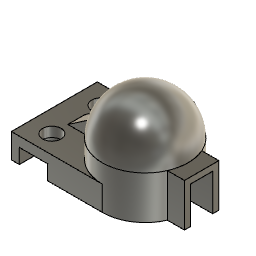
drawing_8 v1 (Autodesk Fusion 360 design; units mm, degrees)
Autodesk Fusion 360 part; units mm, degrees
box "BoxPrimitive1" add length 70 width 74 height 20 placed x (0, -1, 0) y (1, 0, 0) z (0, 0, 1) at (-30, 30, 0)
sketch "Sketch2" plane through (0, 0, 20) normal (0, 0, 1) x (-1, 0, 0)
  line L0 (30, 40) -> (-44, 40)
  line L1 (-44, 40) -> (-44, -30)
  line L2 (-44, -30) -> (30, -30)
  line L3 (30, -30) -> (30, 40)
  circle A0 centre (12, -15) radius 7.5
  circle A1 centre (12, 25) radius 7.5
  point P0 (30, -15)
  point P1 (30, 25)
  point P2 (12, -30)
  point P3 (12, -15)
  point P4 (12, 25)
  dimension "d9" = 15
  dimension "d10" = 15
  constraint coincident P3 A0.centre
  constraint coincident P4 A1.centre
  measures "d9" diameter of A0
  measures "d10" diameter of A1
extrude "Extrude1" cut sketch "Sketch2" against normal blind 378 contours A0 | A1
sketch "Sketch3" plane through (0, 0, 0) normal (0, 0, -1) x (1, 0, 0)
  circle A0 centre (-12, -15) radius 7.5
  circle A1 centre (-12, 25) radius 7.5
  line L0 (44, 40) -> (-30, 40)
  line L1 (-30, 40) -> (-30, -30)
  line L2 (-30, -30) -> (44, -30)
  line L3 (44, -30) -> (44, 40)
  line L4 (-0.5, 25) -> (-0.5, 40)
  line L5 (-0.5, 40) -> (-23.5, 40)
  line L6 (-23.5, 40) -> (-23.5, 25)
  line L7 (-23.5, -15) -> (-23.5, -30)
  line L8 (-23.5, -30) -> (-0.5, -30)
  line L9 (-0.5, -30) -> (-0.5, -15)
  arc A2 (-0.5, -15) -> (-23.5, -15) centre (-12, -15) ccw
  arc A3 (-23.5, 25) -> (-0.5, 25) centre (-12, 25) ccw
  dimension "d13" = 23
  dimension "d14" = 23
  dimension "d15" = 23
  dimension "d16" = 23
  constraint concentric A1 A3
  constraint concentric A0 A2
  constraint coincident L0 L4.end
  constraint tangent L4 A3
  constraint perpendicular L0 L4
  constraint perpendicular L4 L5
  constraint tangent L7 A2
  constraint coincident L2 L8.end
  constraint tangent L9 A2
  measures "d13" diameter of A3
  measures "d14" diameter of A2
  measures "d15" distance of L4.end L5.end
  measures "d16" distance of L7.end L8.end
extrude "Extrude2" cut sketch "Sketch3" against normal blind 12 contours L0 L4 L5 L6 A3 | L2 L7 L8 L9 A2
sketch "Sketch4" plane through (0, 0, 20) normal (0, 0, 1) x (-1, 0, 0)
  circle A0 centre (12, -15) radius 7.5
  circle A1 centre (12, 25) radius 7.5
  line L0 (30, 40) -> (-44, 40)
  line L1 (-44, -30) -> (30, -30)
  line L2 (30, -30) -> (30, 40)
  circle A2 centre (-44, 5) radius 35
  point P0 (-44, 5)
  constraint coincident P0 A2.centre
  constraint coincident L1.start A2
extrude "Extrude3" add sketch "Sketch4" along normal blind 15 and the other way blind 20 contours A2
sketch "Sketch5" plane through (0, 0, 35) normal (0, 0, 1) x (-1, 0, 0)
  circle A0 centre (-44, 5) radius 35
sketch "Sketch6" plane through (0, 0, 35) normal (0, 0, 1) x (-1, 0, 0)
  circle A0 centre (-44, 5) radius 35
  dimension "d23" = 70
  measures "d23" diameter of A0
sphere "SpherePrimitive1" add diameter 70 placed x (-1, 0, 0) y (0, -1, 0) z (0, 0, 1) at (44, -5, 35)
sketch "Sketch8" plane through (0, 30, 0) normal (0, 1, 0) x (-1, 0, 0)
  line L0 (0.5, 0) -> (0.5, 12)
  line L1 (0.5, 12) -> (23.5, 12)
  line L2 (23.5, 12) -> (23.5, 0)
  line L3 (23.5, 0) -> (30, 0)
  line L4 (30, 0) -> (30, 20)
  line L5 (30, 20) -> (-44, 20)
  line L6 (-44, 20) -> (-44, 0)
  line L7 (-44, 0) -> (0.5, 0)
  line L8 (-34, 50) -> (-54, 50)
  line L9 (-54, 50) -> (-54, 30)
  line L10 (-54, 30) -> (-34, 30)
  line L11 (-34, 30) -> (-34, 50)
  line L12 (-34, 50) -> (-54, 30) construction
  line L13 (-54, 50) -> (-34, 30) construction
  point P0 (-44, 40)
  point P1 (-44, 40)
  dimension "d26" = 20
  dimension "d27" = 20
  constraint horizontal L8
  constraint perpendicular L8 L9
  constraint parallel L8 L10
  constraint parallel L9 L11
  constraint coincident L12 P1
  constraint coincident L13 P1
  constraint coincident P1 P0
  measures "d26" distance of L9.end L10.end
  measures "d27" distance of L8.end L9.end
extrude "Extrude4" cut sketch "Sketch8" against normal blind 15 contours L8 L9 L10 L11
sketch "Sketch9" plane through (0, 0, 0) normal (0, 0, -1) x (1, 0, 0)
  line L0 (44, 40) -> (-0.5, 40)
  line L1 (-0.5, 40) -> (-0.5, 25)
  arc A0 (-23.5, 25) -> (-0.5, 25) centre (-12, 25) ccw
  line L2 (-23.5, 25) -> (-23.5, 40)
  line L3 (-23.5, 40) -> (-30, 40)
  line L4 (-30, 40) -> (-30, -30)
  line L5 (-30, -30) -> (-23.5, -30)
  line L6 (-23.5, -30) -> (-23.5, -15)
  arc A1 (-0.5, -15) -> (-23.5, -15) centre (-12, -15) ccw
  line L7 (-0.5, -15) -> (-0.5, -30)
  line L8 (-0.5, -30) -> (44, -30)
  arc A2 (44, -30) -> (44, 40) centre (44, 5) ccw
  circle A3 centre (44, 5) radius 28
extrude "Extrude5" cut sketch "Sketch9" against normal blind 35 contours A3
sketch "Sketch10" plane through (0, 0, 35) normal (0, 0, -1) x (1, 0, 0)
  line L0 (34, -21.1534) -> (34, -15)
  line L1 (34, -15) -> (54, -15)
  line L2 (54, -15) -> (54, -21.1534)
  arc A0 (54, -21.1534) -> (34, -21.1534) centre (44, 5) ccw
  circle A1 centre (44, 5) radius 28
  constraint concentric A0 A1
sphere "SpherePrimitive2" cut diameter 56 placed x (1, 0, 0) y (0, -1, 0) z (0, 0, -1) at (44, -5, 35)
sketch "Sketch12" plane through (0, 0, 20) normal (0, 0, 1) x (-1, 0, 0)
  arc A0 (-44, -30) -> (-44, 40) centre (-44, 5) ccw
  line L0 (-44, -30) -> (30, -30)
  line L1 (30, -30) -> (30, 40)
  line L2 (30, 40) -> (-44, 40)
  circle A1 centre (12, -15) radius 7.5
  circle A2 centre (12, 25) radius 7.5
  line L3 (12, 5) -> (12, -2)
  line L4 (12, -2) -> (12, 5)
  line L5 (12, 5) -> (12, 12)
  line L6 (12, -2) -> (-11.2915, -2)
  line L7 (-11.2915, -2) -> (-11.2915, 12)
  line L8 (-11.2915, 12) -> (12, 12)
  point P0 (30, 5)
  constraint midpoint L1 P0
  constraint perpendicular L3 L6
  constraint perpendicular L6 L7
  constraint perpendicular L7 L8
extrude "Extrude6" add sketch "Sketch12" along normal blind 15 contours A0 L6 L7 L8 | A0 L3 L4 L5 L6 L8
sketch "Sketch13" plane through (0, 2, 0) normal (0, 1, 0) x (-1, 0, 0)
  line L0 (-9.7071, 35) -> (-9.7071, 20)
  line L1 (-9.7071, 20) -> (12, 20)
  line L2 (12, 20) -> (12, 35)
  line L3 (12, 35) -> (-9.7071, 35)
  line L4 (12, 20) -> (-10, 35)
  constraint coincident L1.end L2.start
extrude "Extrude7" cut sketch "Sketch13" against normal blind 20 contours L0 L2 L3 L4
sketch "Sketch14" plane through (0, 0, 0) normal (0, 0, -1) x (1, 0, 0)
  circle A0 centre (44, 5) radius 28
  line L0 (44, 40) -> (-0.5, 40)
  line L1 (-0.5, 40) -> (-0.5, 25)
  arc A1 (-23.5, 25) -> (-0.5, 25) centre (-12, 25) ccw
  line L2 (-23.5, 25) -> (-23.5, 40)
  line L3 (-23.5, 40) -> (-30, 40)
  line L4 (-30, 40) -> (-30, -30)
  line L5 (-30, -30) -> (-23.5, -30)
  line L6 (-23.5, -30) -> (-23.5, -15)
  arc A2 (-0.5, -15) -> (-23.5, -15) centre (-12, -15) ccw
  line L7 (-0.5, -15) -> (-0.5, -30)
  line L8 (-0.5, -30) -> (44, -30)
  arc A3 (44, -30) -> (44, 40) centre (44, 5) ccw
  line L9 (-30, 5) -> (79, 5)
  line L10 (79, 5) -> (90, 5)
  line L11 (90, 5) -> (90, 19)
  line L12 (90, 19) -> (90, 5)
  line L13 (90, 5) -> (90, -9)
  line L14 (90, -9) -> (73.8174, -9)
  line L15 (73.8174, -9) -> (73.8174, 19)
  line L16 (73.8174, 19) -> (90, 19)
  line L17 (90, 19) -> (90, -9)
  constraint midpoint L4 L9.start
  constraint midpoint A3 L9.end
  constraint parallel L9 L10
  constraint perpendicular L10 L11
  constraint perpendicular L10 L13
  constraint horizontal L14
  constraint vertical L15
  constraint horizontal L16
  constraint vertical L17
extrude "Extrude8" add sketch "Sketch14" against normal blind 35 contours A3 L9 L15 L16 | A3 L9 L14 L15 | A3 L10 L13 L14 L17 | A3 L10 L11 L12 L16 L17
sketch "Sketch15" plane through (90, 0, 0) normal (1, 0, 0) x (0, 1, 0)
  line L0 (-19, 0) -> (9, 0)
  line L1 (9, 0) -> (9, 35)
  line L2 (9, 35) -> (-19, 35)
  line L3 (-19, 35) -> (-19, 0)
  line L4 (-5, 0) -> (-14, 0)
  line L5 (-5, 0) -> (4, 0)
  line L6 (-14, 0) -> (4, 0)
  line L7 (4, 0) -> (4, 30)
  line L8 (4, 30) -> (-14, 30)
  line L9 (-14, 30) -> (-14, 0)
  point P0 (-5, 0)
  dimension "d48" = 30
  constraint midpoint L0 P0
  constraint coincident P0 L4.start
  constraint perpendicular L3 L4
  constraint perpendicular L3 L5
  constraint horizontal L6
  constraint vertical L7
  constraint horizontal L8
  constraint vertical L9
  measures "d48" distance of L4.end L8.end
extrude "Extrude9" cut sketch "Sketch15" against normal blind 21 contours L0 L4 L5 L6 L7 L8 L9
